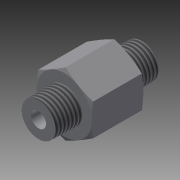
# Autodesk Inventor part: Pneumatic_VIAIR_Fitting
Saved by Autodesk Inventor 2018 (Build 220112000, 112)
## iProperties
Created: 2011-11-29
Part Number: Pneumatic_VIAIR_Fitting
Material: Generic
Document SubType Name: Modeling
Designer: Phillip
Density: 1 g/cm^3
Appearance: Default
Author: Phillip
Autodesk Inventor part; units mm, degrees
ref_plane "YZ Plane" through (0, 0, 0) normal (1, 0, 0) x (0, 1, 0)
sketch "Sketch1" plane through (0, 0, 0) normal (0, 0, 1) x (1, 0, 0)
  circle A0 centre (-12.8329, -29.5246) radius 6.35
  line L0 (-6.0325, -33.4508) -> (-12.8329, -37.377)
  line L1 (-12.8329, -37.377) -> (-19.6333, -33.4508)
  line L2 (-19.6333, -33.4508) -> (-19.6333, -25.5984)
  line L3 (-19.6333, -25.5984) -> (-12.8329, -21.6722)
  line L4 (-12.8329, -21.6722) -> (-6.0325, -25.5984)
  line L5 (-6.0325, -25.5984) -> (-6.0325, -33.4508)
  circle A1 centre (-12.8329, -29.5246) radius 4.3656
  circle A2 centre (-12.8329, -29.5246) radius 6.35
  circle A3 centre (-12.8329, -29.5246) radius 6.8004
  line L6 (-12.8329, -21.6722) -> (-12.8329, -22.7242) construction
  dimension "d36" = 13.6008
  dimension "d37" = 1.052
  constraints: 14 end point, 3 centre point, 2 coincident, 1 concentric, 1 parallel, 1 vertical, 1 vertical alignment, 16 other
  measures "d37" distance of L3.end L6.end
extrude "Extrusion1" add sketch "Sketch1" along normal blind 12.7 contours A0 | L0 A3 L5 | L0 L1 A3 | A3 | A3 L4 L5 | L1 L2 A3 | A3 L3 L4 | L2 L3 A3 | A1
ref_plane "Work Plane1" through (-12.8329, -37.377, 0) normal (-1, 0, 0) x (0, 0, 1)
extrude "Extrusion3" add sketch "Sketch1" against normal blind 6.35 draft -1.783 contours A1
thread "Thread2" size "1/8" designation "1/8 - 27 NPT" standard "NPT for PVC Pipe and Fitting" length 9.9568
sketch "Sketch6" plane through (0, 0, 12.7) normal (0, 0, 1) x (1, 0, 0)
  circle A0 centre (-12.8329, -29.5246) radius 6.35 projected
  point P0 (0, 0)
hole "Hole2" at (-12.8329, -29.5246, 12.7) direction (0, 0, -1) diameter 3.302 end through all
sketch "Sketch7" plane through (0, 0, 12.7) normal (0, 0, 1) x (1, 0, 0)
  circle A0 centre (-12.8329, -29.5246) radius 1.651 projected
  circle A1 centre (-12.8329, -29.5246) radius 4.3656 projected
  point P0 (0, 0)
extrude "Extrusion4" add sketch "Sketch7" along normal blind 6.35 draft -1.783
thread "Thread3" size "1/8" designation "1/8 - 27 NPT" standard "NPT for PVC Pipe and Fitting" length 9.9568
sketch "Sketch8" plane through (-12.8329, -37.377, 0) normal (-1, 0, 0) x (0, 0, 1)
  line L0 (12.7, 14.6507) -> (12.3564, 15.7048)
  line L1 (12.3564, 15.7048) -> (12.7, 14.6507)
  line L2 (12.3564, 15.7048) -> (12.7, 15.7048)
  line L3 (12.7, 15.7048) -> (12.7, 14.6507)
  line L4 (12.7, 15.7048) -> (12.7, 11.7786) projected
  line L5 (16.6116, 7.8524) -> (-10.7696, 7.8524) projected
  point P0 (0, 37.377)
  point P1 (-6.858, -1.905)
  dimension "d38" = 1.0541
  constraints: 8 end point, 2 collinear
  measures "d38" distance from line of L0.start L2
revolve "Revolution3" cut sketch "Sketch8" angle 360 about axis through (-12.8329, -29.5246, 0) along (0, 0, -1)
ref_plane "Work Plane4" through (-12.8329, -29.5246, 6.35) normal (0, 0, 1) x (1, 0, 0)
mirror "Mirror4" about plane through (-12.8329, -29.5246, 6.35) normal (0, 0, 1) of "Revolution3"
body "Solid1"
